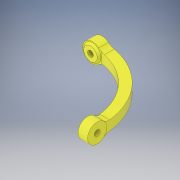
# Autodesk Inventor part: Link
Saved by Autodesk Inventor 2019 (Build 230136000, 136)
## iProperties
Created: 2022-07-05
Part Number: Link
Material: Generic
Document SubType Name: Modeling
Designer: zreik
Density: 1 g/cm^3
Appearance: Smooth - Yellow
width: 35.000 mm
height: 35.000 mm
Author: zreik
Autodesk Inventor part; units mm, degrees
ref_plane "XZ Plane" through (0, 0, 0) normal (0, 1, 0) x (-1, 0, 0)
ref_plane "XY Plane" through (0, 0, 0) normal (0, 0, 1) x (1, 0, 0)
sketch "Sketch1" plane through (0, 0, 0) normal (0, 0, 1) x (1, 0, 0)
  circle A0 centre (0, 0) radius 5
  dimension "d0" = 10
  constraints: 1 centre point, 1 coincident
  measures "d0" diameter of A0
extrude "Extrusion1" add sketch "Sketch1" along normal blind 5
sketch "Sketch2" plane through (0, 0, 0) normal (1, 0, 0) x (0, 1, 0)
  line L0 (-2.5, 5) -> (2.5, 5)
  line L1 (2.5, 5) -> (2.5, 0)
  line L2 (2.5, 0) -> (-2.5, 0)
  line L3 (-2.5, 0) -> (-2.5, 5)
  line L4 (-2.5, 5) -> (2.5, 0) construction
  line L5 (2.5, 5) -> (-2.5, 0) construction
  line L6 (-5, 0) -> (5, 0) projected
  point P0 (0, 0)
  point P1 (0, 2.5)
  dimension "d3" = 2.5
  dimension "d4" = 0
  dimension "d5" = 5
  dimension "d6" = 5
  constraints: 12 end point, 2 midpoint, 2 parallel, 1 horizontal, 1 perpendicular
  measures "d3" distance from line of L6 point (0, 2.5)
  measures "d4" horizontal distance of point (0, 0) point (0, 2.5)
  measures "d5" distance of L0.end L1.end
  measures "d6" distance of L1.end L2.end
sketch "Sketch3" plane through (0, 0, 0) normal (0, 1, 0) x (-1, 0, 0)
  arc A0 (-35, 37.5) -> (-5, 2.5) centre (0.4167, 37.5) ccw
  line L0 (-5, 2.5) -> (0, 2.5)
  line L1 (-35, 37.5) -> (-35, 42.5)
  point P0 (0, 0)
  dimension "d10" = 35
  dimension "d14" = 2.5
  dimension "d15" = 5
  dimension "d17" = 5
  dimension "d24" = 5
  dimension "d68" = 35
  dimension "d69" = 0
  constraints: 4 end point, 2 point on circle, 1 centre point, 1 horizontal, 1 vertical
  measures "d10" horizontal distance of L1.start point (0, 0)
  measures "d14" vertical distance of point (0, 0) L0.start
  measures "d15" horizontal distance of L0.start point (0, 0)
  measures "d17" distance of L0.start L0.end
  measures "d24" distance of L1.start L1.end
  measures "d68" vertical distance of L0.start L1.start
  measures "d69" vertical distance of A0.centre L1.start
sweep "Sweep1" add profiles "Sketch2" path "Sketch3" path curves L0 A0 L1
ref_plane "Work Plane1" through (35, 0, 0) normal (1, 0, 0) x (0, 1, 0)
sketch "Sketch4" plane through (35, 0, 0) normal (1, 0, 0) x (0, 1, 0)
  circle A0 centre (0, 40) radius 5
  point P0 (0, 0)
  dimension "d27" = 10
  dimension "d28" = 40
  dimension "d29" = 0
  constraints: 1 centre point
  measures "d27" diameter of A0
  measures "d28" distance of A0.centre point (0, 0)
  measures "d29" horizontal distance of point (0, 0) A0.centre
extrude "Extrusion2" add sketch "Sketch4" along normal mid plane 5
fillet "Fillet1" radius 5 6 edges at (36.2279, -2.5, 35.6699) (33.75, -2.5, 35.6699) (4.3301, -2.5, 2.5) (4.3301, 2.5, 2.5) (33.75, 2.5, 35.6699) (36.2279, 2.5, 35.6699)
sketch "Sketch10" plane through (0, 0, 5) normal (0, 0, 1) x (1, 0, 0)
  circle A0 centre (0, 0) radius 1.5
  arc A1 (3.3072, 3.75) -> (3.3072, -3.75) centre (0, 0) ccw projected
  dimension "d49" = 3
  constraints: 1 centre point, 1 concentric
  measures "d49" diameter of A0
sketch "Sketch11" plane through (32.5, 0, 40) normal (-1, 0, 0) x (0, 0, 1)
  circle A0 centre (0, 0) radius 1.5
  circle A1 centre (0, 0) radius 5 projected
  point P0 (-40, 0)
  point P1 (-3.3072, -3.75)
  point P2 (-3.3072, 3.75)
  dimension "d50" = 3
  constraints: 1 centre point, 1 concentric
  measures "d50" diameter of A0
extrude "Extrusion8" cut sketch "Sketch11" against normal through all contours A0
extrude "Extrusion9" cut sketch "Sketch10" against normal through all
sketch "Sketch12" plane through (32.5, 0, 40) normal (1, 0, 0) x (0, 0, -1)
  circle A0 centre (0, 0) radius 2.5
  circle A1 centre (0, 0) radius 1.5
  circle A2 centre (0, 0) radius 1.5 projected
  point P0 (40, 0)
  dimension "d55" = 3
  dimension "d56" = 5
  constraints: 2 centre point, 1 coincident, 1 concentric
  measures "d55" diameter of A1
  measures "d56" diameter of A0
extrude "Extrusion10" add sketch "Sketch12" against normal blind 1
chamfer "Chamfer1" distance 1 angle 45 1 edges at (32.5, 0, 42.5)
sketch "Sketch13" plane through (0, 0, 5) normal (0, 0, 1) x (1, 0, 0)
  circle A0 centre (0, 0) radius 3.5
  circle A1 centre (0, 0) radius 1.5 projected
  dimension "d62" = 7
  constraints: 1 centre point, 1 concentric
  measures "d62" diameter of A0
extrude "Extrusion11" add sketch "Sketch13" along normal blind 1
chamfer "Chamfer2" distance 1 angle 45 1 edges at (-3.5, 0, 5)
equation "\"d10\" = width"
equation "\"d68\" = height"
equation "\"d26\" = d10"
equation "\"width\" = 35"
equation "\"height\" = 35"
body "Solid1"
